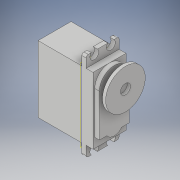
# Autodesk Inventor part: HS-322HD
Saved by Autodesk Inventor 2017 (Build 210142000, 142)
## iProperties
Created: 2017-02-21
Part Number: HS-322HD
Material: Generic
Document SubType Name: Modeling
Designer: kingb
Density: 1 g/cm^3
Appearance: Default
Author: kingb
Autodesk Inventor part; units mm, degrees
ref_plane "YZ Plane" through (0, 0, 0) normal (1, 0, 0) x (0, 1, 0)
ref_plane "XZ Plane" through (0, 0, 0) normal (0, 1, 0) x (-1, 0, 0)
ref_plane "XY Plane" through (0, 0, 0) normal (0, 0, 1) x (1, 0, 0)
sketch "Sketch1" plane through (0, 0, 0) normal (0, 0, 1) x (1, 0, 0)
  line L0 (0, 0) -> (33.02, 0)
  line L1 (33.02, 0) -> (33.02, 40.005)
  line L2 (33.02, 40.005) -> (0, 40.005)
  line L3 (0, 40.005) -> (0, 0)
  dimension "d0" = 33.02
  dimension "d1" = 40.005
  constraints: 8 end point, 2 parallel, 1 horizontal, 1 perpendicular
  measures "d0" distance of L2.end L1.end
  measures "d1" distance of L1.end L0.end
extrude "Extrusion1" add sketch "Sketch1" along normal mid plane 19.812
ref_plane "Work Plane1" through (26.289, 0, 9.906) normal (-1, 0, 0) x (0, 0, 1)
sketch "Sketch2" plane through (26.289, 0, 9.906) normal (-1, 0, 0) x (0, 0, 1)
  line L0 (-19.812, 40.005) -> (0, 40.005) projected
  line L1 (-19.812, 0) -> (0, 0) projected
  line L2 (-9.906, 40.005) -> (0, 40.005)
  line L3 (0, 40.005) -> (0, 46.609)
  line L4 (-9.906, 46.609) -> (-9.906, 44.323)
  arc A0 (-6.7754, 46.609) -> (-3.1052, 46.609) centre (-4.9403, 44.6913) ccw
  line L5 (0, 44.6913) -> (-2.286, 44.6913)
  line L6 (-4.9403, 40.005) -> (-4.9403, 42.037)
  line L7 (-9.906, 40.005) -> (-9.2583, 40.005)
  line L8 (-9.2583, 40.005) -> (-9.2583, 44.323)
  line L9 (-9.2583, 44.323) -> (-9.906, 44.323)
  line L10 (-9.906, 44.323) -> (-9.906, 40.005)
  line L11 (0, 46.609) -> (-3.1052, 46.609)
  line L12 (-6.7754, 46.609) -> (-9.906, 46.609)
  line L13 (-9.906, 40.005) -> (-19.812, 40.005)
  line L14 (-19.812, 40.005) -> (-19.812, 46.609)
  arc A1 (-16.7068, 46.609) -> (-13.0366, 46.609) centre (-14.8717, 44.6913) ccw
  line L15 (-19.812, 44.6913) -> (-17.526, 44.6913)
  line L16 (-14.8717, 40.005) -> (-14.8717, 42.037)
  line L17 (-10.5537, 40.005) -> (-10.5537, 44.323)
  line L18 (-10.5537, 44.323) -> (-9.906, 44.323)
  line L19 (-19.812, 46.609) -> (-16.7068, 46.609)
  line L20 (-13.0366, 46.609) -> (-9.906, 46.609)
  line L21 (0, 0) -> (0, 40.005) projected
  line L22 (-19.812, 40.005) -> (-19.812, 0) projected
  line L23 (0, 20.0025) -> (-19.812, 20.0025) construction
  line L24 (-19.812, 0) -> (0, 0)
  line L25 (0, 0) -> (0, -6.604)
  arc A2 (-3.1052, -6.604) -> (-6.7754, -6.604) centre (-4.9403, -4.6863) ccw
  line L26 (-9.2583, 0) -> (-9.2583, -4.318)
  line L27 (-9.2583, -4.318) -> (-9.906, -4.318)
  line L28 (0, -6.604) -> (-3.1052, -6.604)
  line L29 (-6.7754, -6.604) -> (-9.906, -6.604)
  line L30 (-19.812, -6.604) -> (-16.7068, -6.604)
  line L31 (-19.812, 0) -> (-19.812, -6.604)
  arc A3 (-13.0366, -6.604) -> (-16.7068, -6.604) centre (-14.8717, -4.6863) ccw
  line L32 (-9.906, 0) -> (-19.812, 0)
  line L33 (-10.5537, 0) -> (-10.5537, -4.318)
  line L34 (-10.5537, -4.318) -> (-9.906, -4.318)
  line L35 (-13.0366, -6.604) -> (-9.906, -6.604)
  dimension "d5" = 6.604
  dimension "d6" = 2.286
  dimension "d7" = 2.032
  dimension "d8" = 0.6477
  dimension "d9" = 4.318
  dimension "d11" = 4.318
  constraints: 64 end point, 24 symmetric about line, 12 point on circle, 5 parallel, 4 centre point, 4 point on line, 3 horizontal, 3 midpoint, 3 perpendicular, 2 line through centre, 3 other
  measures "d5" distance of L0.end L3.end
  measures "d6" distance of L5.start L5.end
  measures "d7" distance of L6.start L6.end
  measures "d8" distance of L4.end L8.end
  measures "d9" distance of L8.end L7.end
  measures "d11" horizontal distance of A0.centre L8.end
extrude "Extrusion2" add sketch "Sketch2" against normal blind 2.54 contours L14 L15 A1 L16 L0 | L16 A1 L20 L4 L18 L17 L0 | L14 L19 A1 L15 | L1 L33 L34 L27 L26 L25 L28 A2 L29 L35 A3 L30 L31 | L17 L18 L10 L0 | L1 L26 L27 L34 L33 | L10 L9 L8 L0 | L8 L9 L4 L12 A0 L6 L0 | L6 A0 L5 L3 L0 | L5 A0 L11 L3
fillet "Fillet1" radius 1.27 4 edges at (27.559, 46.609, 9.906) (27.559, 46.609, -9.906) (27.559, -6.604, 9.906) (27.559, -6.604, -9.906)
sketch "Sketch3" plane through (33.02, 0, 9.906) normal (1, 0, 0) x (0, 0, -1)
  line L0 (1.016, 5.715) -> (18.796, 5.715)
  line L1 (18.796, 5.715) -> (18.796, 31.115)
  line L2 (9.906, 40.005) -> (9.906, 40.005)
  line L3 (1.016, 31.115) -> (1.016, 5.715)
  line L4 (19.812, 40.005) -> (0, 40.005) construction
  line L5 (0, 0) -> (0, 40.005) construction
  arc A0 (9.906, 40.005) -> (1.016, 31.115) centre (9.906, 31.115) ccw
  arc A1 (18.796, 31.115) -> (9.906, 40.005) centre (9.906, 31.115) ccw
  line L6 (9.906, 5.715) -> (9.906, 3.429) construction
  arc A2 (5.461, 5.715) -> (9.906, 3.429) centre (9.906, 8.8935) ccw
  arc A3 (9.906, 3.429) -> (14.351, 5.715) centre (9.906, 8.8935) ccw
  point P0 (9.906, 0)
  point P1 (18.796, 40.005)
  point P2 (1.016, 40.005)
  dimension "d15" = 17.78
  dimension "d16" = 34.29
  dimension "d17" = 1.016
  dimension "d18" = 8.89
  dimension "d19" = 2.286
  dimension "d20" = 8.89
  dimension "d21" = 4.445
  constraints: 10 end point, 8 point on circle, 7 point on line, 4 centre point, 4 tangent, 2 line through centre, 2 parallel, 1 concentric, 1 horizontal, 1 midpoint, 1 perpendicular, 1 vertical
  measures "d15" distance of point (1.016, 40.005) point (18.796, 40.005)
  measures "d16" distance of point (18.796, 40.005) L0.end
  measures "d17" distance between parallel lines of L5 L3
  measures "d18" radius of A0
  measures "d19" distance of L6.start L6.end
  measures "d20" distance of A2.start A3.end
  measures "d21" distance of L6.start A2.start
extrude "Extrusion3" add sketch "Sketch3" along normal blind 2.794
sketch "Sketch4" plane through (35.814, 0, 9.906) normal (1, 0, 0) x (0, 0, -1)
  arc A0 (18.796, 31.115) -> (1.016, 31.115) centre (9.906, 31.115) ccw projected
  circle A1 centre (9.906, 31.115) radius 4.445
  point P0 (9.906, 0)
  dimension "d24" = 8.89
  constraints: 1 centre point, 1 coincident
  measures "d24" diameter of A1
extrude "Extrusion4" add sketch "Sketch4" along normal blind 4.826
sketch "Sketch5" plane through (40.64, 31.115, 0) normal (1, 0, 0) x (0, 0, -1)
  circle A0 centre (0, 0) radius 11.8745
  circle A1 centre (0, 0) radius 2.9845
  point P0 (0, -31.115)
  dimension "d27" = 23.749
  dimension "d28" = 5.969
  constraints: 2 centre point, 1 coincident
  measures "d27" diameter of A0
  measures "d28" diameter of A1
extrude "Extrusion5" add sketch "Sketch5" along normal blind 1.905
body "Solid1"
